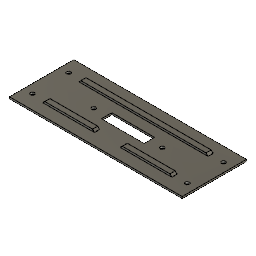
smmb_top (Autodesk Fusion 360 design; units mm, degrees)
Autodesk Fusion 360 part; units mm, degrees
sketch "Sketch1" plane through (0, 0, 0) normal (0, 0, 1) x (1, 0, 0)
  line L0 (0, 0) -> (134, 0)
  line L1 (134, 0) -> (134, 50)
  line L2 (134, 50) -> (0, 50)
  line L3 (0, 50) -> (0, 0)
  circle A0 centre (7, 39) radius 1.55
  circle A1 centre (7, 11) radius 1.55
  circle A2 centre (127, 39) radius 1.55
  circle A3 centre (127, 11) radius 1.55
  line L4 (83.5, 21) -> (50.5, 21)
  line L5 (50.5, 21) -> (50.5, 29)
  line L6 (50.5, 29) -> (83.5, 29)
  line L7 (83.5, 29) -> (83.5, 21)
  line L8 (83.5, 21) -> (50.5, 29) construction
  line L9 (50.5, 21) -> (83.5, 29) construction
  line L10 (0, 25) -> (134, 25) construction
  circle A4 centre (40.5, 25) radius 1.55
  circle A5 centre (93.5, 25) radius 1.55
  line L11 (7, 11) -> (127, 11) construction
  line L12 (117, 9) -> (17, 9)
  line L13 (17, 9) -> (17, 13)
  line L14 (17, 13) -> (117, 13)
  line L15 (117, 13) -> (117, 9)
  line L16 (117, 9) -> (17, 13) construction
  line L17 (17, 9) -> (117, 13) construction
  line L18 (117, 41) -> (17, 41)
  line L19 (17, 41) -> (17, 37)
  line L20 (17, 37) -> (117, 37)
  line L21 (117, 37) -> (117, 41)
  line L22 (77, 9) -> (57, 9)
  line L23 (57, 9) -> (57, 13)
  line L24 (57, 13) -> (77, 13)
  line L25 (77, 13) -> (77, 9)
  line L26 (77, 9) -> (57, 13) construction
  line L27 (57, 9) -> (77, 13) construction
  point P0 (67, 25)
  point P1 (67, 11)
  point P2 (67, 11)
  dimension "d1" = 134
  dimension "d2" = 50
  dimension "d3" = 3.1
  dimension "d4" = 11
  dimension "d5" = 7
  dimension "d6" = 3.1
  dimension "d7" = 3.1
  dimension "d8" = 3.1
  dimension "d9" = 7
  dimension "d10" = 11
  dimension "d11" = 11
  dimension "d12" = 7
  dimension "d13" = 7
  dimension "d14" = 11
  dimension "d15" = 33
  dimension "d16" = 8
  dimension "d17" = 21
  dimension "d18" = 50.5
  dimension "d19" = 3.1
  dimension "d20" = 26.5
  dimension "d21" = 3.1
  dimension "d22" = 26.5
  dimension "d28" = 4
  constraint horizontal L0
  constraint vertical L1
  constraint horizontal L2
  constraint vertical L3
  constraint coincident L0.start L3.end
  constraint perpendicular L4 L5
  constraint parallel L4 L6
  constraint parallel L5 L7
  constraint horizontal L4
  constraint coincident L8 P0
  constraint coincident L9 P0
  constraint midpoint L3 L10.start
  constraint midpoint L1 L10.end
  constraint coincident L10 A4.centre
  constraint coincident L10 A5.centre
  constraint coincident A1.centre L11.start
  constraint coincident A3.centre L11.end
  constraint perpendicular L12 L13
  constraint parallel L12 L14
  constraint parallel L13 L15
  constraint horizontal L12
  constraint coincident L16 P2
  constraint coincident L17 P2
  constraint midpoint L11 P2
  constraint symmetric L10 L12.start L18.start
  constraint symmetric L10 L12.end L18.end
  constraint symmetric L10 L13.end L19.end
  constraint symmetric L10 L14.end L20.end
  constraint perpendicular L22 L23
  constraint parallel L22 L24
  constraint parallel L23 L25
  constraint horizontal L22
  constraint coincident L12 L22.start
  constraint coincident L26 P2
  constraint coincident L27 P2
  constraint coincident P2 P1
  measures "d1" distance of L0.start L0.end
  measures "d2" distance of L0.start L2.end
  measures "d3" diameter of A0
  measures "d4" distance of L2 A0.centre
  measures "d5" distance of L3 A0.centre
  measures "d6" diameter of A1
  measures "d7" diameter of A3
  measures "d8" diameter of A2
  measures "d9" distance of L3 A1.centre
  measures "d10" distance of L0 A1.centre
  measures "d11" distance of L2 A2.centre
  measures "d12" distance of L1 A2.centre
  measures "d13" distance of L1 A3.centre
  measures "d14" distance of L0 A3.centre
  measures "d15" distance of L5.end L6.end
  measures "d16" distance of L4.end L5.end
  measures "d17" distance of L2 L6
  measures "d18" distance of L3 L5
  measures "d19" diameter of A4
  measures "d20" distance of P0 A4.centre
  measures "d21" diameter of A5
  measures "d22" distance of P0 A5.centre
  measures "d28" distance of L22.end L23.end
extrude "Extrude1" add sketch "Sketch1" along normal blind 1.5 contours L0 L1 L2 L3 | L12 L14 L15 L25 | L12 L14 L22 L23 L24 L25 | L12 L13 L14 L23 | L18 L19 L20 L21
extrude "Extrude2" add sketch "Sketch1" along normal blind 3 contours L12 L14 L15 L25 | L12 L13 L14 L23 | L18 L19 L20 L21
chamfer "Chamfer1" distance 1.5 angle 45 4 edges at (117, 11, 3) (117, 39, 3) (17, 39, 3) (17, 11, 3)
chamfer "Chamfer2" distance 1.5 angle 45 2 edges at (57, 11, 3) (77, 11, 3)
equation "d6 = d3"
equation "d7 = d3"
equation "d8 = d3"
equation "d9 = d5"
equation "d10 = d4"
equation "d11 = d4"
equation "d12 = d5"
equation "d13 = d5"
equation "d14 = d4"
equation "d19 = d3"
equation "d21 = d3"
equation "d22 = d20"
